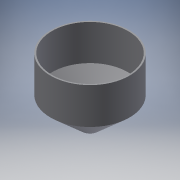
# Autodesk Inventor part: LargerWidefieldCone_v3
Saved by Autodesk Inventor 2016 (Build 200138000, 138)
## iProperties
Created: 2014-12-01
Part Number: LargerWidefieldCone_v3
Material: Generic
Document SubType Name: Sheet Metal
Designer: ChurchlandLab
Density: 1 g/cm^3
Sheet Metal Rule: Default
Appearance: Default
Author: ChurchlandLab
Autodesk Inventor part; units mm, degrees
ref_plane "YZ Plane" through (0, 0, 0) normal (1, 0, 0) x (0, 1, 0)
ref_plane "XZ Plane" through (0, 0, 0) normal (0, 1, 0) x (-1, 0, 0)
ref_plane "XY Plane" through (0, 0, 0) normal (0, 0, 1) x (1, 0, 0)
sketch "Sketch1" plane through (0, 0, 0) normal (0, 0, 1) x (1, 0, 0)
  line L0 (0, 0) -> (0, 68.58)
  line L1 (0, 68.58) -> (40.64, 68.58)
  line L2 (40.64, 30.48) -> (6.35, 0)
  line L3 (6.35, 0) -> (0, 0)
  line L4 (40.64, 68.58) -> (40.64, 30.48)
  dimension "d1" = 40.64
  dimension "d2" = 6.35
  dimension "d6" = 90
  dimension "d21" = 38.1
  dimension "d22" = 30.48
  constraints: 10 end point, 1 parallel, 1 perpendicular, 1 vertical
  measures "d1" distance of L1.end L0.end
  measures "d2" distance of L2.end L0.start
  measures "d6" angle of L1 L4
  measures "d21" distance of L1.end L2.start
  measures "d22" vertical distance of L2.end L2.start
revolve "Revolution1" add sketch "Sketch1" angle 360 about axis through (0, 0, 0) along (0, 1, 0)
shell "Shell1" thickness 1.5 outward yes removed faces 2 at (-10.0721, 68.58, 13.6928) at (-1.8127, 0, 0.4771)
sketch "Sketch2" plane through (0, 0, 0) normal (0, -1, 0) x (1, 0, 0)
  line L0 (6.2865, -0.8255) -> (7.9502, -0.8255)
  line L1 (7.9502, -0.8255) -> (7.9502, 0.8255)
  line L2 (7.9502, 0.8255) -> (6.2865, 0.8255)
  line L3 (6.2865, 0.8255) -> (6.2865, -0.8255)
  line L4 (6.2865, -0.8255) -> (7.9502, 0.8255) construction
  line L5 (7.9502, -0.8255) -> (6.2865, 0.8255) construction
  line L6 (0, 1.1822) -> (0, -1.5875) construction
  line L7 (-6.2865, -0.8255) -> (-7.9502, -0.8255)
  line L8 (-7.9502, -0.8255) -> (-7.9502, 0.8255)
  line L9 (-7.9502, 0.8255) -> (-6.2865, 0.8255)
  line L10 (-6.2865, 0.8255) -> (-6.2865, -0.8255)
  line L11 (2.1925, 0) -> (-0.3475, 0) construction
  line L12 (-0.8255, 6.2865) -> (0.8255, 6.2865)
  line L13 (0.8255, 6.2865) -> (0.8255, 7.9502)
  line L14 (0.8255, 7.9502) -> (-0.8255, 7.9502)
  line L15 (-0.8255, 7.9502) -> (-0.8255, 6.2865)
  line L16 (-0.8255, 6.2865) -> (0.8255, 7.9502) construction
  line L17 (0.8255, 6.2865) -> (-0.8255, 7.9502) construction
  line L18 (-0.8255, -6.2865) -> (0.8255, -6.2865)
  line L19 (0.8255, -6.2865) -> (0.8255, -7.9502)
  line L20 (0.8255, -7.9502) -> (-0.8255, -7.9502)
  line L21 (-0.8255, -7.9502) -> (-0.8255, -6.2865)
  line L22 (-0.8255, -6.2865) -> (0.8255, -7.9502) construction
  line L23 (0.8255, -6.2865) -> (-0.8255, -7.9502) construction
  circle A0 centre (0, 0) radius 6.35 projected
  point P0 (0, 0)
  point P1 (7.1183, 0)
  point P2 (-7.1183, 0)
  point P3 (0, 7.1183)
  point P4 (0, -7.1183)
  dimension "d8" = 1.651
  dimension "d9" = 1.6637
  dimension "d11" = 1.6637
  dimension "d12" = 1.651
  dimension "d17" = 0.0635
  dimension "d18" = 0.0635
  constraints: 48 end point, 10 symmetric about line, 6 midpoint, 4 parallel, 2 horizontal, 2 perpendicular, 2 point on line
  measures "d8" distance of L2.end L0.start
  measures "d9" distance of L0.start L0.end
  measures "d11" distance of L14.end L12.start
  measures "d12" distance of L12.start L12.end
  measures "d17" distance edge to line of A0 L12
  measures "d18" distance edge to line of A0 L3
extrude "Extrusion3" cut sketch "Sketch2" against normal blind 1.651 contours L3 L2 A0 L0 | A0 L2 L1 L0 | A0 L21 L18 L19 | L19 L20 L21 A0 | A0 L15 L14 L13 | L13 L12 L15 A0 | A0 L9 L10 L7 | L7 L8 L9 A0
equation "\"BendRadius\" = Thickness"
equation "\"BendReliefWidth\" = Thickness"
equation "\"BendReliefDepth\" = 0.5 * Thickness"
equation "\"CornerReliefSize\" = 4 * Thickness"
equation "\"MinimumRemnant\" = 2 * Thickness"
equation "\"TransitionRadius\" = BendRadius"
equation "\"JacobiRadiusSize\" = BendRadius"
equation "\"GapSize\" = Thickness"
equation "\"Thickness\" = 3.048"
body "Solid1"
